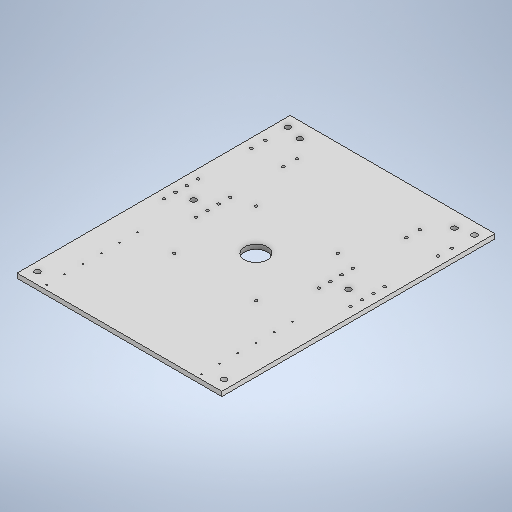
# Autodesk Inventor part: arc
Saved by Autodesk Inventor 2026.1 (Build 301233000, 233)
## iProperties
Created: 2026-05-12
Part Number: arc
Material: Generic
Document SubType Name: Modeling
Designer: chris
Density: 1 g/cm^3
Appearance: Default
Author: chris
Autodesk Inventor part; units mm, degrees
ref_plane "YZ Plane" through (0, 0, 0) normal (1, 0, 0) x (0, 1, 0)
ref_plane "XZ Plane" through (0, 0, 0) normal (0, 1, 0) x (-1, 0, 0)
ref_plane "XY Plane" through (0, 0, 0) normal (0, 0, 1) x (1, 0, 0)
sketch "Sketch1" plane through (0, 0, 0) normal (0, 1, 0) x (-1, 0, 0)
  line L0 (225, 300) -> (-225, 300)
  line L1 (-225, 300) -> (-225, -300)
  line L2 (-225, -300) -> (225, -300)
  line L3 (225, -300) -> (225, 300)
  line L4 (225, 300) -> (-225, -300) construction
  line L5 (-225, 300) -> (225, -300) construction
  point P0 (0, 0)
  dimension "d0" = 450
  dimension "d1" = 600
  constraints: 12 end point, 2 midpoint, 2 parallel, 1 horizontal, 1 perpendicular
  measures "d0" distance of L2.end L1.end
  measures "d1" distance of L1.end L0.end
extrude "Extrusion1" add sketch "Sketch1" along normal blind 10
sketch "Sketch2" plane through (0, 10, 0) normal (0, 1, 0) x (1, 0, 0)
  circle A0 centre (-170, -290) radius 1.5
  circle A1 centre (-170, -250) radius 1.5
  circle A2 centre (-170, -210) radius 1.5
  circle A3 centre (-170, -170) radius 1.5
  circle A4 centre (-170, -90) radius 1.5
  circle A5 centre (-170, -130) radius 1.5
  line L0 (-225, 300) -> (-225, -300) projected
  line L1 (-225, -300) -> (225, -300) projected
  point P0 (0, 0)
  dimension "d4" = 3
  dimension "d5" = 3
  dimension "d6" = 3
  dimension "d7" = 3
  dimension "d8" = 3
  dimension "d9" = 3
  dimension "d10" = 40
  dimension "d11" = 40
  dimension "d12" = 40
  dimension "d13" = 40
  dimension "d14" = 40
  dimension "d15" = 55
  dimension "d16" = 10
  constraints: 6 centre point, 5 vertical alignment
  measures "d4" diameter of A0
  measures "d5" diameter of A1
  measures "d6" diameter of A2
  measures "d7" diameter of A3
  measures "d8" diameter of A4
  measures "d9" diameter of A5
  measures "d10" distance of A1.centre A0.centre
  measures "d11" distance of A2.centre A1.centre
  measures "d12" distance of A3.centre A2.centre
  measures "d13" distance of A5.centre A3.centre
  measures "d14" distance of A4.centre A5.centre
  measures "d15" distance from line of A0.centre L0
  measures "d16" distance from line of L1 A0.centre
extrude "Extrusion2" cut sketch "Sketch2" against normal blind 10
sketch "Sketch3" plane through (0, 10, 0) normal (0, 1, 0) x (1, 0, 0)
  circle A0 centre (0, 0) radius 25
  circle A1 centre (90, -90) radius 3
  circle A2 centre (90, 90) radius 3
  circle A3 centre (-90, 90) radius 3
  circle A4 centre (-90, -90) radius 3
  dimension "d19" = 50
  dimension "d20" = 6
  dimension "d21" = 6
  dimension "d22" = 6
  dimension "d23" = 6
  dimension "d24" = 90
  dimension "d25" = 90
  dimension "d26" = 90
  dimension "d27" = 90
  dimension "d28" = 90
  dimension "d29" = 90
  dimension "d30" = 90
  dimension "d31" = 90
  constraints: 5 centre point, 1 coincident
  measures "d19" diameter of A0
  measures "d20" diameter of A1
  measures "d21" diameter of A2
  measures "d22" diameter of A3
  measures "d23" diameter of A4
  measures "d24" horizontal distance of A3.centre point (0, 0)
  measures "d25" horizontal distance of A4.centre point (0, 0)
  measures "d26" horizontal distance of A1.centre point (0, 0)
  measures "d27" horizontal distance of A2.centre point (0, 0)
  measures "d28" horizontal distance of A2.centre point (0, 0)
  measures "d29" horizontal distance of point (0, 0) A3.centre
  measures "d30" horizontal distance of point (0, 0) A4.centre
  measures "d31" horizontal distance of A1.centre point (0, 0)
extrude "Extrusion3" cut sketch "Sketch3" against normal blind 10
mirror "Mirror1" about plane through (0, 0, 0) normal (1, 0, 0) of "Extrusion2"
sketch "Sketch4" plane through (0, 10, 0) normal (0, 1, 0) x (1, 0, 0)
  circle A0 centre (-205, 275) radius 6
  line L0 (225, 300) -> (-225, 300) projected
  line L1 (-225, 300) -> (-225, -300) projected
  point P0 (0, 0)
  dimension "d34" = 12
  dimension "d35" = 25
  dimension "d36" = 20
  constraints: 1 centre point
  measures "d34" diameter of A0
  measures "d35" distance from line of L0 A0.centre
  measures "d36" distance from line of L1 A0.centre
extrude "Extrusion4" cut sketch "Sketch4" against normal blind 10
mirror "Mirror2" about plane through (0, 0, 0) normal (1, 0, 0) of "Extrusion4"
mirror "Mirror3" about plane through (0, 0, 0) normal (0, 0, 1) of "Extrusion4", "Mirror2"
sketch "Sketch5" plane through (0, 10, 0) normal (0, 1, 0) x (1, 0, 0)
  circle A0 centre (-205, 225) radius 3
  circle A1 centre (-205, 195) radius 3
  circle A2 centre (-205, 78) radius 3
  circle A3 centre (-205, 53) radius 3
  circle A4 centre (-205, 28) radius 3
  circle A5 centre (-205, 3) radius 3
  circle A6 centre (-135, 225) radius 3
  circle A7 centre (-135, 195) radius 3
  circle A8 centre (-135, 78) radius 3
  circle A9 centre (-135, 53) radius 3
  circle A10 centre (-135, 28) radius 3
  circle A11 centre (-135, 3) radius 3
  line L0 (-225, 300) -> (-225, -300) projected
  circle A12 centre (-170, 33) radius 6
  line L1 (225, 300) -> (-225, 300) projected
  circle A13 centre (-170, 266) radius 6
  point P0 (0, 0)
  dimension "d39" = 6
  dimension "d40" = 6
  dimension "d41" = 6
  dimension "d42" = 6
  dimension "d43" = 6
  dimension "d44" = 6
  dimension "d45" = 6
  dimension "d46" = 6
  dimension "d47" = 6
  dimension "d48" = 6
  dimension "d49" = 6
  dimension "d50" = 6
  dimension "d51" = 20
  dimension "d52" = 90
  dimension "d53" = 12
  dimension "d54" = 55
  dimension "d55" = 75
  dimension "d56" = 105
  dimension "d57" = 25
  dimension "d58" = 272
  dimension "d59" = 25
  dimension "d60" = 25
  dimension "d61" = 267
  dimension "d62" = 12
  dimension "d63" = 55
  dimension "d64" = 34
  constraints: 14 centre point, 10 vertical alignment, 6 horizontal alignment
  measures "d39" diameter of A0
  measures "d40" diameter of A1
  measures "d41" diameter of A2
  measures "d42" diameter of A3
  measures "d43" diameter of A4
  measures "d44" diameter of A5
  measures "d45" diameter of A6
  measures "d46" diameter of A7
  measures "d47" diameter of A8
  measures "d48" diameter of A9
  measures "d49" diameter of A10
  measures "d50" diameter of A11
  measures "d51" distance from line of L0 A0.centre
  measures "d52" distance from line of L0 A6.centre
  measures "d53" diameter of A12
  measures "d54" distance from line of L0 A12.centre
  measures "d55" distance from line of L1 A0.centre
  measures "d56" distance from line of A1.centre L1
  measures "d57" distance of A10.centre A9.centre
  measures "d58" distance from line of A4.centre L1
  measures "d59" distance of A2.centre A3.centre
  measures "d60" distance of A5.centre A4.centre
  measures "d61" distance from line of A12.centre L1
  measures "d62" diameter of A13
  measures "d63" distance from line of L0 A13.centre
  measures "d64" distance from line of L1 A13.centre
extrude "Extrusion5" cut sketch "Sketch5" against normal blind 10
mirror "Mirror4" about plane through (0, 0, 0) normal (1, 0, 0) of "Extrusion5"
body "Solid1"
